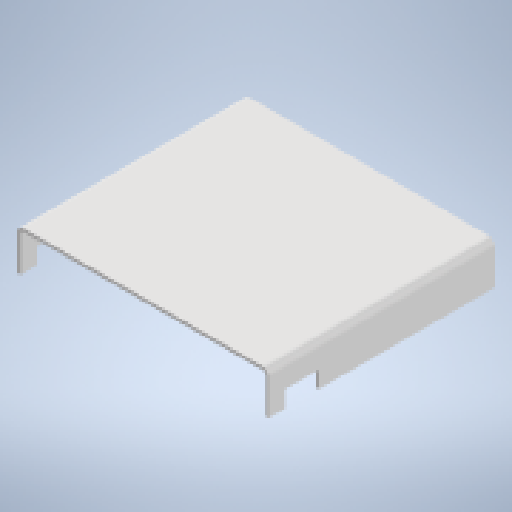
# Autodesk Inventor part: ДМС 310 швеллер лотка
Saved by Autodesk Inventor 2024.2 (Build 282272000, 272)
## iProperties
Created: 2024-05-13
Part Number: ДМС 310 швеллер лотка
Material: Generic
Document SubType Name: Sheet Metal
Designer: admin
Density: 1 g/cm^3
Appearance: Default
Sheet Metal Rule: Default
Author: admin
Autodesk Inventor part; units mm, degrees
ref_plane "YZ Plane" through (0, 0, 0) normal (1, 0, 0) x (0, 1, 0)
ref_plane "XZ Plane" through (0, 0, 0) normal (0, 1, 0) x (-1, 0, 0)
ref_plane "XY Plane" through (0, 0, 0) normal (0, 0, 1) x (1, 0, 0)
sketch "Sketch1" plane through (0, 0, 0) normal (0, 0, 1) x (1, 0, 0)
  line L0 (-75, 0) -> (75, 0)
  line L1 (75, 0) -> (75, -135)
  line L2 (75, -135) -> (-75, -135)
  line L3 (-75, -135) -> (-75, 0)
  point P0 (0, 0)
  point P1 (0, 0)
  dimension "d0" = 150
  dimension "d1" = 135
  measures "d0" distance of L1.end L2.end
  measures "d1" distance of L0.end L1.end
extrude "Plate1" add sketch "Sketch1" along normal blind 2
sketch "Sketch2" plane through (73, -135, 2) normal (1, 0, 0) x (0, 1, 0)
  line L0 (135, 0) -> (0, 0)
  line L1 (0, 0) -> (0, -25)
  line L2 (0, -25) -> (135, -25)
  line L3 (135, -25) -> (135, 0)
  constraints: 6 end point, 1 horizontal, 1 perpendicular, 1 vertical
edge flange "Flange1" height 25 angle 90 thickness 2 bend radius 2 thickness toward (1, 0, 0) relief straight relief width 2 relief depth 1 corner gap 2 corner form 0 edges at (75, -67.5, 0) (-75, -67.5, 0) wall of the first edge with corners at (73, 0, 2) (73, -135, 2) (73, -135, -23) (73, 0, -23)
bend "Bend1"
corner "Corner1"
sketch "Sketch3" plane through (0, 0, 0) normal (1, 0, 0) x (0, 1, 0)
  line L0 (0, -2) -> (-135, -2) projected
  line L1 (-135, -23) -> (-135, -2) projected
  line L2 (0, -23) -> (-135, -23) projected
  line L3 (0, -2) -> (0, -23) projected
  line L4 (-125, -23) -> (-105, -23)
  line L5 (-105, -23) -> (-105, -13)
  line L6 (-105, -13) -> (-125, -13)
  line L7 (-125, -13) -> (-125, -23)
  point P0 (0, 0)
  point P1 (-105, -23)
  point P2 (-125, -18)
  dimension "d13" = 20
  dimension "d14" = 10
  dimension "d17" = 10
  constraints: 8 end point, 2 parallel, 1 horizontal, 1 midpoint, 1 perpendicular, 1 point on line
  measures "d13" distance of L6.end L5.end
  measures "d14" distance of L5.end L4.end
  measures "d17" distance from line of L1 point (-125, -18)
extrude "Extrusion1" cut sketch "Sketch3" along normal through all both and the other way through all contours L2 L7 L6 L5
equation "\"d2\" = Thickness"
equation "\"d3\" = BendReliefWidth"
equation "\"d4\" = BendReliefDepth"
equation "\"d5\" = MinimumRemnant"
equation "\"d6\" = TransitionRadius"
equation "\"d9\" = BendRadius"
equation "\"d10\" = CornerReliefSize"
equation "\"d11\" = GapSize"
equation "\"d12\" = JacobiRadiusSize"
equation "\"GapSize\" = Thickness"
equation "\"BendRadius\" = Thickness"
equation "\"MinimumRemnant\" = 2 * Thickness"
equation "\"BendReliefDepth\" = 0.5 * Thickness"
equation "\"BendReliefWidth\" = Thickness"
equation "\"CornerReliefSize\" = 4 * Thickness"
equation "\"JacobiRadiusSize\" = BendRadius"
equation "\"TransitionRadius\" = BendRadius"
equation "\"Thickness\" = 2"
body "Solid1"
